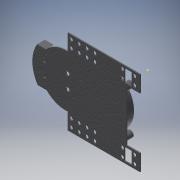
# Autodesk Inventor part: BaseChassis
Saved by Autodesk Inventor 2016 (Build 200138000, 138)
## iProperties
Created: 2016-02-17
Part Number: BaseChassis
Material: Generic
Document SubType Name: Modeling
Designer: mkepler
Density: 1 g/cm^3
Appearance: Default
Author: mkepler
Autodesk Inventor part; units mm, degrees
ref_plane "YZ Plane" through (0, 0, 0) normal (1, 0, 0) x (0, 1, 0)
ref_plane "XZ Plane" through (0, 0, 0) normal (0, 1, 0) x (-1, 0, 0)
ref_plane "XY Plane" through (0, 0, 0) normal (0, 0, 1) x (1, 0, 0)
sketch "Sketch1" plane through (0, 0, 0) normal (0, 1, 0) x (-1, 0, 0)
  line L0 (0, 0) -> (0, -24)
  line L1 (0, 0) -> (106, 0)
  line L2 (106, 0) -> (106, -24)
  line L3 (0, -24) -> (20, -24)
  line L4 (20, -24) -> (20, -100)
  line L5 (20, -100) -> (0, -100)
  line L6 (0, -100) -> (0, -124)
  line L7 (0, -124) -> (106, -124)
  line L8 (106, -124) -> (106, -100)
  arc A0 (106, -100) -> (106, -24) centre (109.0526, -62) ccw
  dimension "d0" = 24
  dimension "d2" = 106
  dimension "d3" = 24
  dimension "d4" = 20
  dimension "d5" = 76
  dimension "d6" = 24
  dimension "d7" = 106
  dimension "d8" = 24
  constraints: 18 end point, 4 vertical, 3 horizontal, 2 perpendicular, 2 point on circle, 1 centre point
  measures "d0" distance of L0.start L0.end
  measures "d2" distance of L0.start L1.end
  measures "d3" distance of L1.end L2.end
  measures "d4" distance of L0.end L3.end
  measures "d5" distance of L3.end L4.end
  measures "d6" distance of L5.end L6.end
  measures "d7" distance of L6.end L7.end
  measures "d8" distance of L7.end L8.end
extrude "Extrusion1" add sketch "Sketch1" along normal blind 1.5
sketch "Sketch2" plane through (0, 1.5, 0) normal (0, 1, 0) x (1, 0, 0)
  circle A0 centre (-8, 6) radius 2.5
  line L0 (0, 0) -> (0, 24) projected
  line L1 (-8, 6) -> (-8, 18)
  line L2 (-8, 18) -> (-26, 18)
  line L3 (-26, 18) -> (-26, 6)
  circle A1 centre (-26, 6) radius 2.5
  circle A2 centre (-26, 18) radius 2.5
  circle A3 centre (-8, 18) radius 2.5
  line L4 (-20, 24) -> (-20, 100) projected
  line L5 (-20, 62) -> (-147.458, 62)
  circle A4 centre (-8, 118) radius 2.5
  circle A5 centre (-26, 118) radius 2.5
  circle A6 centre (-26, 106) radius 2.5
  circle A7 centre (-8, 106) radius 2.5
  line L6 (-106, 0) -> (0, 0) projected
  dimension "d11" = 5
  dimension "d12" = 8
  dimension "d15" = 18
  dimension "d16" = 12
  dimension "d17" = 5
  dimension "d18" = 5
  dimension "d19" = 5
  dimension "d31" = 6
  constraints: 8 centre point, 8 end point, 7 symmetric about line, 6 coincident, 2 horizontal, 1 midpoint, 1 perpendicular, 1 vertical, 4 other
  measures "d11" diameter of A0
  measures "d12" distance from line of L0 L1.start
  measures "d15" distance of L1.end L2.end
  measures "d16" distance of L2.end L3.end
  measures "d17" diameter of A1
  measures "d18" diameter of A2
  measures "d19" diameter of A3
  measures "d31" distance from line of L6 L1.start
hole "Hole1" at (-26, 1.5, -6) at (-26, 1.5, -18) at (-8, 1.5, -6) at (-8, 1.5, -18) at (-26, 1.5, -106) at (-26, 1.5, -118) at (-8, 1.5, -106) at (-8, 1.5, -118) direction (0, -1, 0) diameter 5 depth 8 tip angle 118
sketch "Sketch3" plane through (0, 1.5, 0) normal (0, 1, 0) x (1, 0, 0)
  line L0 (-22.75, 3) -> (-11.75, 3)
  line L1 (-11.75, 3) -> (-11.75, 21)
  line L2 (-11.75, 21) -> (-22.75, 21)
  line L3 (-22.75, 21) -> (-22.75, 3)
  circle A0 centre (-26, 6) radius 2.5 projected
  circle A1 centre (-26, 18) radius 2.5 projected
  line L4 (-26, 6) -> (-26, 18)
  line L5 (-106, 0) -> (0, 0) projected
  circle A2 centre (-8, 6) radius 2.5 projected
  line L6 (-20, 24) -> (-20, 100) projected
  line L7 (-20, 62) -> (-40.9657, 62)
  line L8 (-22.75, 121) -> (-11.75, 121)
  line L9 (-11.75, 121) -> (-11.75, 103)
  line L10 (-11.75, 103) -> (-22.75, 103)
  line L11 (-22.75, 103) -> (-22.75, 121)
  dimension "d27" = 11
  dimension "d28" = 18
  dimension "d29" = 3.25
  dimension "d30" = 3
  constraints: 20 end point, 4 symmetric about line, 2 horizontal, 2 parallel, 1 midpoint, 1 perpendicular, 1 vertical
  measures "d27" distance of L2.end L1.end
  measures "d28" distance of L1.end L0.end
  measures "d29" distance between parallel lines of L4 L3
  measures "d30" distance between parallel lines of L5 L0
extrude "Extrusion2" cut sketch "Sketch3" against normal blind 1.5 contours L3 L2 L1 L0 | L8 L9 L10 L11
sketch "Sketch4" plane through (0, 1.5, 0) normal (0, 1, 0) x (1, 0, 0)
  circle A0 centre (-101, 6) radius 2.5
  line L0 (-106, 24) -> (-106, 0) projected
  line L1 (-106, 0) -> (0, 0) projected
  circle A1 centre (-101, 17.5) radius 2.5
  circle A2 centre (-89.5, 17.5) radius 2.5
  circle A3 centre (-89.5, 6) radius 2.5
  line L2 (-89.5, 6) -> (-83.75, 6)
  line L3 (-83.75, 0) -> (-83.75, 6.5764)
  circle A4 centre (-66.5, 6) radius 2.5
  circle A5 centre (-66.5, 17.5) radius 2.5
  circle A6 centre (-78, 17.5) radius 2.5
  circle A7 centre (-78, 6) radius 2.5
  line L4 (-20, 24) -> (-20, 100) projected
  line L5 (-20, 62) -> (-53, 62)
  circle A8 centre (-101, 118) radius 2.5
  circle A9 centre (-101, 106.5) radius 2.5
  circle A10 centre (-89.5, 106.5) radius 2.5
  circle A11 centre (-89.5, 118) radius 2.5
  circle A12 centre (-66.5, 106.5) radius 2.5
  circle A13 centre (-78, 106.5) radius 2.5
  circle A14 centre (-78, 118) radius 2.5
  circle A15 centre (-66.5, 118) radius 2.5
  dimension "d34" = 5
  dimension "d35" = 5
  dimension "d36" = 6
  dimension "d37" = 5
  dimension "d38" = 11.5
  dimension "d39" = 5
  dimension "d40" = 11.5
  dimension "d41" = 5
  dimension "d42" = 5.75
  constraints: 16 centre point, 12 symmetric about line, 6 end point, 2 horizontal, 1 midpoint, 1 point on line, 1 vertical, 12 other
  measures "d34" diameter of A0
  measures "d35" distance from line of L0 A0.centre
  measures "d36" distance from line of A0.centre L1
  measures "d37" diameter of A1
  measures "d38" distance of A1.centre A0.centre
  measures "d39" diameter of A2
  measures "d40" distance of A2.centre A1.centre
  measures "d41" diameter of A3
  measures "d42" distance of L2.start L2.end
hole "Hole2" at (-101, 1.5, -118) at (-101, 1.5, -106.5) at (-89.5, 1.5, -106.5) at (-89.5, 1.5, -118) at (-78, 1.5, -118) at (-78, 1.5, -106.5) at (-66.5, 1.5, -106.5) at (-66.5, 1.5, -118) at (-66.5, 1.5, -17.5) at (-66.5, 1.5, -6) at (-78, 1.5, -6) at (-78, 1.5, -17.5) at (-89.5, 1.5, -17.5) at (-89.5, 1.5, -6) at (-101, 1.5, -6) at (-101, 1.5, -17.5) direction (0, -1, 0) diameter 5 depth 8 tip angle 118
sketch "Sketch5" plane through (0, 1.5, 0) normal (0, 1, 0) x (1, 0, 0)
  arc A0 (-106, 100) -> (-106, 24) centre (-109.0526, 62) ccw projected
  line L0 (-106, 24) -> (-106, 0) projected
  line L1 (-106, 24) -> (-106, 100)
  line L2 (-106, 62) -> (-106, 72)
  line L3 (-106, 62) -> (-106, 52)
  line L4 (-106, 72) -> (-140, 72)
  circle A1 centre (-140, 72) radius 2.75
  circle A2 centre (-106, 72) radius 2.75
  circle A3 centre (-106, 52) radius 2.75
  circle A4 centre (-140, 52) radius 2.75
  point P0 (0, 0)
  dimension "d56" = 10
  dimension "d57" = 10
  dimension "d58" = 34
  dimension "d60" = 5.5
  dimension "d61" = 5.5
  dimension "d62" = 5.5
  dimension "d63" = 5.5
  constraints: 8 end point, 4 centre point, 3 coincident, 2 point on line, 1 horizontal, 1 midpoint, 1 vertical
  measures "d56" distance of L2.start L2.end
  measures "d57" distance of L2.start L3.end
  measures "d58" distance of L2.end L4.end
  measures "d60" diameter of A1
  measures "d61" diameter of A2
  measures "d62" diameter of A3
  measures "d63" diameter of A4
hole "Hole3" at (-140, 1.5, -52) at (-140, 1.5, -72) at (-106, 1.5, -72) at (-106, 1.5, -52) direction (0, -1, 0) diameter 5.5 depth 8 tip angle 118
sketch "Sketch6" plane through (0, 1.5, 0) normal (0, 1, 0) x (1, 0, 0)
  arc A0 (-106, 100) -> (-106, 24) centre (-109.0526, 62) ccw projected
  line L0 (-106, 24) -> (-106, 16)
  line L1 (-106, 24) -> (-106, 0) projected
  arc A1 (-149.9608, 88.4033) -> (-150.8331, 37) centre (-109.0526, 62) ccw
  line L2 (-106, 24) -> (-106, 37)
  line L3 (-137.8331, 37) -> (-150.8331, 37)
  line L4 (-136.5514, 88.4033) -> (-149.9608, 88.4033)
  line L5 (-20, 24) -> (-20, 100) projected
  line L6 (-22.75, 21) -> (-22.75, 3) projected
  circle A2 centre (-26, 18) radius 2.5 projected
  circle A3 centre (-26, 106) radius 2.5 projected
  circle A4 centre (-25.5, 30.5) radius 5
  circle A5 centre (-25.5, 93.5) radius 5
  line L7 (-22.75, 103) -> (-11.75, 103) projected
  arc A6 (-45, 24) -> (-45, 100) centre (-61.38, 62) ccw
  line L8 (-45, 24) -> (-53, 24)
  line L9 (-45, 100) -> (-53, 100)
  arc A7 (-53, 24) -> (-53, 100) centre (-61.1047, 62) ccw
  point P0 (0, 0)
  dimension "d71" = 8
  dimension "d72" = 13
  dimension "d80" = 10
  dimension "d82" = 25
  dimension "d85" = 8
  dimension "d103" = 10
  dimension "d104" = 13
  constraints: 12 end point, 8 point on circle, 5 centre point, 3 horizontal, 1 concentric, 1 parallel, 1 point on line, 1 tangent, 1 vertical
  measures "d71" distance of L0.start L0.end
  measures "d72" distance of L0.start L2.end
  measures "d80" diameter of A4
  measures "d82" distance of L5.start L8.start
  measures "d85" distance of L8.start L8.end
  measures "d103" diameter of A5
  measures "d104" distance of L3.start L3.end
extrude "Extrusion3" add sketch "Sketch6" along normal blind 10 contours A0 L3 A1 L4 | A4 | A5 | L8 A7 L9 A6
sketch "Sketch14" plane through (0, 11.5, 0) normal (0, 1, 0) x (1, 0, 0)
  circle A0 centre (-152.6674, 62) radius 3
  circle A1 centre (-25.5, 30.5) radius 5 projected
  circle A2 centre (-25.5, 30.5) radius 3
  circle A3 centre (-25.5, 93.5) radius 5 projected
  circle A4 centre (-25.5, 93.5) radius 3
  line L0 (-20, 24) -> (-20, 62) projected
  line L1 (-20, 24) -> (-106.5908, 24)
  line L2 (-20, 100) -> (-106.5908, 100)
  line L3 (-20, 100) -> (0, 100) projected
  line L4 (-20, 24) -> (-20, 100)
  arc A5 (-149.9608, 88.4033) -> (-150.8331, 37) centre (-109.0526, 62) ccw projected
  line L5 (-157.7415, 62) -> (-157.7415, 0)
  line L6 (-106, 0) -> (0, 0) projected
  line L7 (-36, 0) -> (-36, 24)
  line L8 (0, 0) -> (0, 24) projected
  point P0 (-37.3564, 24)
  dimension "d112" = 6
  dimension "d113" = 6
  dimension "d114" = 6
  dimension "d125" = 63
  dimension "d126" = 6.5
  dimension "d127" = 6.5
  dimension "d128" = 137.7415
  dimension "d129" = 36
  constraints: 10 end point, 3 centre point, 2 coincident, 2 horizontal, 2 point on line, 2 vertical, 1 point on circle, 1 tangent
  measures "d112" diameter of A0
  measures "d113" diameter of A2
  measures "d114" diameter of A4
  measures "d125" distance of A4.centre A2.centre
  measures "d126" distance from line of L1 A2.centre
  measures "d127" distance from line of L2 A4.centre
  measures "d128" distance of L5.start L0.end
  measures "d129" distance between parallel lines of L7 L8
hole "Hole5" at (-152.6674, 11.5, -62) at (-25.5, 11.5, -93.5) at (-25.5, 11.5, -30.5) direction (0, -1, 0) diameter 6 depth 10
sketch "Sketch16" plane through (0, 1.5, 0) normal (0, -1, 0) x (1, 0, 0)
  line L0 (-150.8331, -37) -> (-137.8331, -37) projected
  line L1 (-137.8331, -37) -> (-150.8331, -37)
  line L2 (-136.5514, -88.4033) -> (-149.9608, -88.4033) projected
  line L3 (-149.9608, -88.4033) -> (-137.1257, -88.4033)
  arc A0 (-155.2887, -47.678) -> (-155.8682, -47.7805) centre (-155.5152, -48.0874) ccw
  arc A1 (-150.8331, -37) -> (-149.9608, -88.4033) centre (-109.0526, -62) ccw projected
  arc A2 (-137.8331, -37) -> (-136.5514, -88.4033) centre (-109.0526, -62) ccw projected
  arc A3 (-137.8331, -37) -> (-137.8331, -37) centre (-109.0526, -62) ccw
  point P0 (0, 0)
  constraints: 4 end point, 2 point on circle, 1 centre point, 1 collinear, 1 point on line, 4 other
extrude "Extrusion6" add sketch "Sketch16" along normal blind 1.5 contours L0 A2 L2 A1
sketch "Sketch17" plane through (0, 11.5, 0) normal (0, 1, 0) x (1, 0, 0)
  line L0 (-152.6674, 62) -> (-157.7415, 62)
  point P0 (0, 0)
  constraints: 2 end point, 1 horizontal
equation "\"d0\" = xl_w2"
equation "\"d2\" = xl_l + batt_l"
equation "\"d3\" = batt_w"
equation "\"d6\" = xl_w2"
equation "\"d7\" = xl_l + batt_l"
equation "\"d8\" = batt_w"
equation "\"d9\" = thickness"
equation "\"d11\" = xl_dia"
equation "\"d15\" = xl_holes_d2"
equation "\"d16\" = xl_holes_d1"
equation "\"d17\" = xl_dia"
equation "\"d18\" = xl_dia"
equation "\"d19\" = xl_dia"
equation "\"d20\" = xl_dia"
equation "\"d28\" = xl_conn_l"
equation "\"d32\" = thickness"
equation "\"d34\" = batt_hole_dia"
equation "\"d37\" = batt_hole_dia"
equation "\"d39\" = batt_hole_dia"
equation "\"d41\" = batt_hole_dia"
equation "\"d43\" = batt_hole_dia"
equation "\"d56\" = 0.5 * cast_hole_sep_w"
equation "\"d57\" = 0.5 * cast_hole_sep_w"
equation "\"d58\" = cast_hole_sep_l"
equation "\"d60\" = cast_dia"
equation "\"d61\" = cast_dia"
equation "\"d62\" = cast_dia"
equation "\"d63\" = cast_dia"
equation "\"d64\" = cast_dia"
equation "\"d86\" = height"
equation "\"d112\" = peg_dia"
equation "\"d113\" = peg_dia"
equation "\"d114\" = peg_dia"
equation "\"d115\" = peg_dia"
equation "\"d122\" = thickness"
equation "\"xl_l\" = 36"
equation "\"xl_w1\" = 21"
equation "\"xl_w2\" = 24"
equation "\"xl_h1\" = 24"
equation "\"xl_h2\" = 26.9"
equation "\"batt_l\" = 70"
equation "\"batt_w\" = 24"
equation "\"xl_dia\" = 5"
equation "\"xl_holes_d1\" = 12"
equation "\"xl_holes_d2\" = 18"
equation "\"xl_conn_l\" = 18"
equation "\"xl_conn_w\" = 11"
equation "\"batt_hole_dia\" = 5"
equation "\"batt_holes_d1\" = 1"
equation "\"batt_holes_d_edge1\" = 4.5"
equation "\"batt_holes_d2_edge\" = 5.5"
equation "\"batt_holes_d3_edge\" = 1"
equation "\"cast_l\" = 44.5"
equation "\"cast_w\" = 30.5"
equation "\"cast_dia\" = 5.5"
equation "\"cast_hole_sep_l\" = 34"
equation "\"height\" = 10"
equation "\"thickness\" = 1.5"
equation "\"peg_dia\" = 6"
equation "\"cast_hole_sep_w\" = 20"
body "Solid1"
